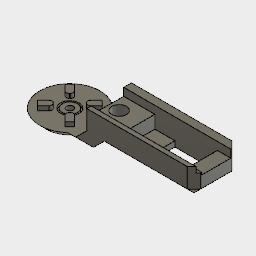
Knee Cross (x4) (Autodesk Fusion 360 design; units mm, degrees)
Autodesk Fusion 360 part; units mm, degrees
sketch "Sketch1" plane through (0, 0, 0) normal (0, 1, 0) x (1, 0, 0)
  circle A0 centre (0, 0) radius 13.5
  line L0 (9.0692, 10) -> (9.0692, -10) construction
  line L1 (9.0692, 10) -> (17.5692, 10)
  line L2 (17.5692, 10) -> (17.5692, -10)
  line L3 (17.5692, -10) -> (9.0692, -10)
  line L4 (9.0692, -10) -> (9.0692, 10)
  dimension "d1" = 27
  dimension "d51" = 8.5
  dimension "d52" = 20
  measures "d1" diameter of A0
  measures "d51" distance of L0.start L1.end
  measures "d52" distance of L0.start L0.end
extrude "Extrude1" add sketch "Sketch1" along normal blind 3 makes body 1
sketch "Sketch2" plane through (0, 3, 0) normal (0, 1, 0) x (-1, 0, 0)
  arc A0 (-9.0692, -10) -> (-9.0692, 10) centre (0, 0) ccw
  circle A1 centre (0, 0) radius 1.5
  line L0 (-9.0692, 10) -> (-17.5692, 10)
  line L1 (-17.5692, 10) -> (-17.5692, -10)
  line L2 (-17.5692, -10) -> (-9.0692, -10)
  dimension "d12" = 3
  measures "d12" diameter of A1
extrude "Extrude2" cut sketch "Sketch2" against normal blind 10 contours A1 bodies 1
sketch "Sketch3" plane through (0, 3, 0) normal (0, 1, 0) x (-1, 0, 0)
  circle A0 centre (0, 0) radius 1.5
  arc A1 (-9.0692, -10) -> (-9.0692, 10) centre (0, 0) ccw
  circle A2 centre (0, 0) radius 3.4
  circle A3 centre (0, 0) radius 4.125
  line L0 (-9.0692, 10) -> (-17.5692, 10)
  line L1 (-17.5692, 10) -> (-17.5692, -10)
  line L2 (-17.5692, -10) -> (-9.0692, -10)
  dimension "d16" = 6.8
  dimension "d17" = 8.25
  measures "d16" diameter of A2
  measures "d17" diameter of A3
extrude "Extrude3" cut sketch "Sketch3" against normal blind 1 contours A3 bodies 1
sketch "Sketch4" plane through (0, 3, 0) normal (0, 1, 0) x (-1, 0, 0)
  arc A0 (-9.0692, -10) -> (-9.0692, 10) centre (0, 0) ccw
  circle A1 centre (0, 0) radius 4.125
  line L0 (0, 0) -> (-7.2478, 7.2478) construction
  line L1 (0, 0) -> (10.5, 0) construction
  line L2 (0, 0) -> (7.2478, -7.2478) construction
  line L3 (0, 0) -> (10.5, 0) construction
  line L4 (0, 0) -> (-7.2478, -7.2478) construction
  line L5 (0, 0) -> (10.5, 0) construction
  line L6 (0, 0) -> (7.2478, 7.2478) construction
  line L7 (-9.0692, 10) -> (-17.5692, 10)
  line L8 (-17.5692, 10) -> (-17.5692, -10)
  line L9 (-17.5692, -10) -> (-9.0692, -10)
  line L10 (-7.2478, -7.2478) -> (-8.3085, -6.1872) construction
  line L11 (-7.2478, 7.2478) -> (-6.1872, 8.3085) construction
  line L12 (7.2478, 7.2478) -> (8.3085, 6.1872) construction
  line L13 (7.2478, -7.2478) -> (6.1872, -8.3085) construction
  line L14 (-8.3085, -6.1872) -> (-6.1872, -8.3085)
  line L15 (-8.3085, -6.1872) -> (-5.3085, -6.1872) construction
  line L16 (-6.1872, -8.3085) -> (-2.6517, -4.773)
  line L17 (-2.6517, -4.773) -> (-4.773, -2.6517)
  line L18 (-4.773, -2.6517) -> (-8.3085, -6.1872)
  line L19 (6.1872, -8.3085) -> (8.3085, -6.1872)
  line L20 (8.3085, -6.1872) -> (4.773, -2.6517)
  line L21 (4.773, -2.6517) -> (2.6517, -4.773)
  line L22 (4.773, -2.6517) -> (7.773, -2.6517) construction
  line L23 (2.6517, -4.773) -> (6.1872, -8.3085)
  line L24 (8.3085, 6.1872) -> (6.1872, 8.3085)
  line L25 (6.1872, 8.3085) -> (2.6517, 4.773)
  line L26 (2.6517, 4.773) -> (4.773, 2.6517)
  line L27 (4.773, 2.6517) -> (8.3085, 6.1872)
  line L28 (-6.1872, 8.3085) -> (-8.3085, 6.1872)
  line L29 (-6.1872, 8.3085) -> (-3.1872, 8.3085) construction
  line L30 (-8.3085, 6.1872) -> (-4.773, 2.6517)
  line L31 (-8.3085, 6.1872) -> (-3.3085, 6.1872) construction
  line L32 (-4.773, 2.6517) -> (-2.6517, 4.773)
  line L33 (-4.773, 2.6517) -> (-1.773, 2.6517) construction
  line L34 (-2.6517, 4.773) -> (-6.1872, 8.3085)
  dimension "d21" = 135
  dimension "d22" = 10.25
  dimension "d23" = 45
  dimension "d24" = 10.25
  dimension "d25" = 135
  dimension "d26" = 10.25
  dimension "d27" = 10.25
  dimension "d107" = 1.5
  dimension "d108" = 1.5
  dimension "d109" = 1.5
  dimension "d110" = 1.5
  dimension "d111" = 45
  dimension "d112" = 3
  dimension "d113" = 5
  dimension "d114" = 3
  dimension "d115" = 3
  dimension "d116" = 5
  dimension "d117" = 135
  dimension "d118" = 3
  dimension "d119" = 3
  dimension "d120" = 5
  dimension "d121" = 3
  dimension "d122" = 135
  dimension "d123" = 3
  dimension "d124" = 45
  dimension "d125" = 5
  dimension "d126" = 45
  dimension "d127" = 3
  measures "d21" angle of L0 L1
  measures "d22" distance of A0.centre L0.end
  measures "d23" angle of L2 L3
  measures "d24" distance of A0.centre L2.end
  measures "d25" angle of L4 L5
  measures "d26" distance of A0.centre L4.end
  measures "d27" distance of A0.centre L6.end
  measures "d107" distance of L4.end L10.end
  measures "d108" distance of L0.end L11.end
  measures "d109" distance of L6.end L12.end
  measures "d110" distance of L2.end L13.end
  measures "d111" angle of L14 L15
  measures "d112" distance of L10.end L14.end
  measures "d113" distance of L14.end L16.end
  measures "d114" distance of L16.end L17.end
  measures "d115" distance of L13.end L19.end
  measures "d116" distance of L19.end L20.end
  measures "d117" angle of L21 L22
  measures "d118" distance of L20.end L21.end
  measures "d119" distance of L12.end L24.end
  measures "d120" distance of L24.end L25.end
  measures "d121" distance of L25.end L26.end
  measures "d122" angle of L28 L29
  measures "d123" distance of L11.end L28.end
  measures "d124" angle of L30 L31
  measures "d125" distance of L28.end L30.end
  measures "d126" angle of L32 L33
  measures "d127" distance of L30.end L32.end
sketch "Sketch5" plane through (0, 3, 0) normal (0, 1, 0) x (-1, 0, 0)
  arc A0 (-9.0692, -10) -> (-9.0692, 10) centre (0, 0) ccw
  line L0 (-9.0692, 10) -> (-17.5692, 10)
  line L1 (-17.5692, 10) -> (-17.5692, -10)
  line L2 (-17.5692, -10) -> (-9.0692, -10)
  circle A1 centre (0, 0) radius 4.125
  line L3 (-17.5692, -10) -> (-65.5692, -10)
  line L4 (-65.5692, -10) -> (-65.5692, 10)
  line L5 (-65.5692, 10) -> (-17.5692, 10)
  line L6 (-17.5692, 10) -> (-17.5692, -10)
  dimension "d53" = 48
  dimension "d54" = 20
  measures "d53" distance of L1.end L3.end
  measures "d54" distance of L1.end L0.end
extrude "Extrude5" add sketch "Sketch5" along normal blind 11.75 separate body contours L1 L3 L4 L5 L6 makes body 2
extrude "Extrude14" add sketch "Sketch4" along normal blind 2 contours L14 L16 L17 L18 | L19 L20 L21 L23 | L24 L25 L26 L27 | L28 L30 L32 L34 bodies 2 1
move_body "MoveBody1" bodies 2 to x (1, 0, 0) y (0, 1, 0) z (0, 0, 1) at (0, 1.875, 0)
fillet "Fillet2" radius 1.35 8 edges at (-4.773, 4, -2.6517) (-2.6517, 4, -4.773) (2.6517, 4, -4.773) (4.773, 4, -2.6517) (4.773, 4, 2.6517) (2.6517, 4, 4.773) (-2.6517, 4, 4.773) (-4.773, 4, 2.6517) on bodies 1
sketch "Sketch6" plane through (0, 0, 10) normal (0, 0, 1) x (1, 0, 0)
  line L0 (9.0692, 0) -> (17.5692, 0)
  line L1 (17.5692, 0) -> (17.5692, 3)
  line L2 (17.5692, 3) -> (9.0692, 3)
  line L3 (9.0692, 3) -> (9.0692, 0)
  line L4 (17.5692, 0) -> (22.789, 5.2199)
  line L5 (17.5692, 0) -> (24.9512, 0) construction
  line L6 (17.5692, 0) -> (17.5692, 4.875)
  line L7 (22.4442, 4.875) -> (17.5692, 4.875)
  point P0 (17.5692, 4.875)
  dimension "d58" = 45
  dimension "d59" = 7.382
  measures "d58" angle of L4 L5
  measures "d59" distance of L0.end L4.end
extrude "Extrude6" add sketch "Sketch6" against normal blind 20 contours L1 L4 L6 L7 bodies 1 2
sketch "Sketch7" plane through (0, 16.625, 0) normal (0, 1, 0) x (-1, 0, 0)
  line L0 (-17.5692, 10) -> (-65.5692, 10)
  line L1 (-65.5692, 10) -> (-65.5692, -10)
  line L2 (-65.5692, -10) -> (-17.5692, -10)
  line L3 (-17.5692, -10) -> (-17.5692, 10)
  line L4 (-17.5692, -10) -> (-17.5692, -6.5)
  line L5 (-17.5692, -6.5) -> (-65.5692, -6.5)
  line L6 (-65.5692, -6.5) -> (-65.5692, 6.5)
  line L7 (-65.5692, 6.5) -> (-17.5692, 6.5)
  line L8 (-17.5692, 6.5) -> (-17.5692, -6.5)
  dimension "d62" = 3.5
  dimension "d63" = 13
  dimension "d64" = 48
  measures "d62" distance of L2.end L4.end
  measures "d63" distance of L4.end L7.end
  measures "d64" distance of L4.end L5.end
extrude "Extrude7" cut sketch "Sketch7" against normal blind 3.5 contours L1 L3 L5 L6 L7 L8 bodies 1
sketch "Sketch8" plane through (0, 16.625, 0) normal (0, 1, 0) x (-1, 0, 0)
  line L0 (-65.5692, 6.5) -> (-17.5692, 6.5)
  line L1 (-17.5692, 6.5) -> (-17.5692, 10)
  line L2 (-17.5692, 10) -> (-65.5692, 10)
  line L3 (-65.5692, 10) -> (-65.5692, 6.5)
  line L4 (-65.5692, 6.5) -> (-17.5692, 6.5)
  line L5 (-17.5692, 6.5) -> (-17.5692, 8)
  line L6 (-17.5692, 8) -> (-65.5692, 8)
  line L7 (-65.5692, 8) -> (-65.5692, 6.5)
  dimension "d67" = 48
  dimension "d68" = 1.5
  measures "d67" distance of L0.start L0.end
  measures "d68" distance of L0.start L6.end
extrude "Extrude8" cut sketch "Sketch8" against normal blind 2.5 contours L0 L1 L3 L4 L5 L6 L7 bodies 1
sketch "Sketch9" plane through (0, 13.125, 0) normal (0, 1, 0) x (-1, 0, 0)
  line L0 (-17.5692, 6.5) -> (-65.5692, 6.5)
  line L1 (-65.5692, 6.5) -> (-65.5692, -6.5)
  line L2 (-65.5692, -6.5) -> (-17.5692, -6.5)
  line L3 (-17.5692, -6.5) -> (-17.5692, 6.5)
  line L4 (-17.5692, 0) -> (-22.0692, 0) construction
  circle A0 centre (-22.0692, 0) radius 3.25
  dimension "d71" = 4.5
  dimension "d72" = 6.5
  measures "d71" distance of L4.start L4.end
  measures "d72" diameter of A0
extrude "Extrude9" cut sketch "Sketch9" against normal blind 6 contours A0 bodies 1
sketch "Sketch10" plane through (0, 7.125, 0) normal (0, 1, 0) x (-1, 0, 0)
  circle A0 centre (-22.0692, 0) radius 3.25
  circle A1 centre (-22.0692, 0) radius 1.75
  dimension "d78" = 3.5
  measures "d78" diameter of A1
extrude "Extrude10" cut sketch "Sketch10" against normal blind 314 contours A1 bodies 1
sketch "Sketch11" plane through (0, 4.875, 0) normal (0, -1, 0) x (1, 0, 0)
  arc A0 (22.4442, -1.7093) -> (22.4442, 1.7093) centre (22.0692, 0) ccw
  line L0 (22.4442, -1.7093) -> (22.4442, -10)
  line L1 (22.4442, -10) -> (65.5692, -10)
  line L2 (65.5692, -10) -> (65.5692, 10)
  line L3 (65.5692, 10) -> (22.4442, 10)
  line L4 (22.4442, 10) -> (22.4442, 1.7093)
  circle A1 centre (22.0692, 0) radius 3
  dimension "d82" = 6
  measures "d82" diameter of A1
extrude "Extrude11" cut sketch "Sketch11" along normal blind 12 contours A0 L0 L4 A1 | A0 L0 L4 A1 bodies 1
sketch "Sketch12" plane through (0, 13.125, 0) normal (0, 1, 0) x (-1, 0, 0)
  circle A0 centre (-22.0692, 0) radius 3.25
  line L0 (-17.5692, 6.5) -> (-65.5692, 6.5)
  line L1 (-65.5692, 6.5) -> (-65.5692, -6.5)
  line L2 (-65.5692, -6.5) -> (-17.5692, -6.5)
  line L3 (-17.5692, -6.5) -> (-17.5692, 6.5)
  line L4 (-65.5692, -6.5) -> (-59.5692, -6.5) construction
  line L5 (-59.5692, -6.5) -> (-40.5692, -6.5)
  line L6 (-40.5692, -6.5) -> (-40.5692, 6.5)
  line L7 (-40.5692, 6.5) -> (-59.5692, 6.5)
  line L8 (-59.5692, 6.5) -> (-59.5692, -6.5)
  dimension "d86" = 6
  dimension "d87" = 19
  dimension "d88" = 13
  measures "d86" distance of L1.end L4.end
  measures "d87" distance of L4.end L5.end
  measures "d88" distance of L4.end L7.end
extrude "Extrude12" cut sketch "Sketch12" against normal blind 54 contours L0 L2 L5 L6 L7 L8 bodies 1
sketch "Sketch13" plane through (0, 13.125, 0) normal (0, 1, 0) x (-1, 0, 0)
  circle A0 centre (-22.0692, 0) radius 3.25
  line L0 (-40.5692, 6.5) -> (-40.5692, -6.5)
  line L1 (-40.5692, -6.5) -> (-17.5692, -6.5)
  line L2 (-17.5692, -6.5) -> (-17.5692, 6.5)
  line L3 (-17.5692, 6.5) -> (-40.5692, 6.5)
  line L4 (-17.5692, -6.5) -> (-31.5692, -6.5) construction
  line L5 (-31.5692, -6.5) -> (-40.5692, -6.5)
  line L6 (-40.5692, -6.5) -> (-40.5692, 6.5)
  line L7 (-40.5692, 6.5) -> (-31.5692, 6.5)
  line L8 (-31.5692, 6.5) -> (-31.5692, -6.5)
  dimension "d91" = 14
  dimension "d92" = 9
  dimension "d93" = 13
  measures "d91" distance of L1.end L4.end
  measures "d92" distance of L4.end L0.end
  measures "d93" distance of L4.end L7.end
extrude "Extrude13" cut sketch "Sketch13" against normal blind 5.75 contours L0 L1 L3 L5 L6 L7 L8 bodies 1
sketch "Sketch14" plane through (0, 0, 10) normal (0, 0, 1) x (1, 0, 0)
  line L0 (9.0692, 0) -> (17.5692, 0)
  line L1 (17.5692, 0) -> (22.4442, 4.875)
  line L2 (22.4442, 4.875) -> (65.5692, 4.875)
  line L3 (65.5692, 4.875) -> (65.5692, 16.625)
  line L4 (65.5692, 16.625) -> (17.5692, 16.625)
  line L5 (17.5692, 16.625) -> (17.5692, 3)
  line L6 (17.5692, 3) -> (9.0692, 3)
  line L7 (9.0692, 3) -> (9.0692, 0)
  line L8 (22.4442, 4.875) -> (14.4442, 4.875)
  line L9 (17.5692, 4.875) -> (17.5692, 3)
  dimension "d96" = 8
  measures "d96" distance of L1.end L8.end
chamfer "Chamfer6" distance 3 angle 45 5 edges at (44.0067, 4.875, 10) (65.5692, 10.75, 10) (65.5692, 4.875, 0) (65.5692, 10.75, -10) (44.0067, 4.875, -10) on bodies 1
chamfer "Chamfer7" distance 3 angle 45 3 edges at (-13.5, 0, 0) (13.3192, 0, 10) (13.3192, 0, -10) on bodies 1
chamfer "Chamfer8" distance 5 angle 45 1 edges at (17.5692, 3, 0) on bodies 1
boxprimitive "BoxPrimitive1" [suppressed]
chamfer "Chamfer9" [suppressed]
chamfer "Chamfer10" [suppressed]
chamfer "Chamfer11" [suppressed]
chamfer "Chamfer12" [suppressed]
chamfer "Chamfer13" [suppressed]
chamfer "Chamfer14" [suppressed]
delete_face "DeleteFace1" [suppressed]
chamfer "Chamfer15" [suppressed]
chamfer "Chamfer16" [suppressed]
chamfer "Chamfer17" [suppressed]
chamfer "Chamfer18" [suppressed]
delete_face "DeleteFace2" [suppressed]
delete_face "DeleteFace3" [suppressed]
delete_face "DeleteFace4" [suppressed]
chamfer "Chamfer19" [suppressed]
equation "HipSeparation = 8.5 mm"
equation "d9 = BottomThickness"
equation "BottomThickness = 3 mm"
equation "d12 = ScrewHole"
equation "ScrewHole = 3 mm"
equation "HornFit = 1.35 mm"
equation "d51 = HipSeparation"
equation "JointFit = 1.875 mm" comment "this is half the full value"
equation "d71 = HolePosX"
equation "d72 = HoleSize"
equation "HolePosX = 4.5 mm"
equation "d74 = -HoleSeparation"
equation "HoleSeparation = 6 mm"
equation "HoleSize = 6.5 mm"
equation "d78 = SpacerScrewHoleSize"
equation "ScrewHoleSize = 3 mm"
equation "d82 = ScrewHeadSize"
equation "ScrewHeadSize = 6 mm"
equation "ChamferStrength = 5 mm"
equation "Chamfer3 = 3 mm"
equation "d106 = ChamferStrength"
equation "FilletFIT = 1.35 mm"
equation "d131 = FilletFIT"
equation "SpacerScrewHoleSize = 3.5 mm"
